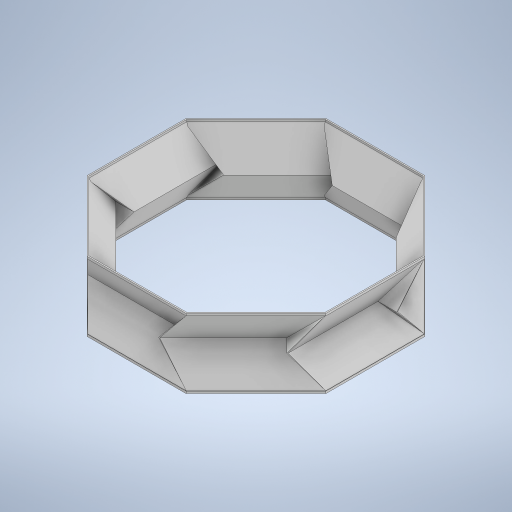
# Autodesk Inventor part: 팔각형 OV-PAM 층 한개
Saved by Autodesk Inventor 2024 (Build 280153000, 153)
## iProperties
Created: 2023-06-16
Part Number: 팔각형 OV-PAM 층 한개
Material: 일반
Document SubType Name: Modeling
Designer: jsw
Density: 1 g/cm^3
Appearance: 기본값
Author: jsw
Autodesk Inventor part; units mm, degrees
ref_plane "YZ Plane" through (0, 0, 0) normal (1, 0, 0) x (0, 1, 0)
ref_plane "XZ Plane" through (0, 0, 0) normal (0, 1, 0) x (-1, 0, 0)
ref_plane "XY Plane" through (0, 0, 0) normal (0, 0, 1) x (1, 0, 0)
sketch "스케치1" plane through (0, 0, 0) normal (0, 1, 0) x (-1, 0, 0)
  line L0 (-65.1838, 27) -> (-27, 65.1838)
  line L1 (-27, 65.1838) -> (27, 65.1838)
  line L2 (27, 65.1838) -> (65.1838, 27)
  line L3 (65.1838, 27) -> (65.1838, -27)
  line L4 (65.1838, -27) -> (27, -65.1838)
  line L5 (27, -65.1838) -> (-27, -65.1838)
  line L6 (-27, -65.1838) -> (-65.1838, -27)
  line L7 (-65.1838, -27) -> (-65.1838, 27)
  line L8 (-27.2485, 65.7838) -> (27.2485, 65.7838)
  line L9 (27.2485, 65.7838) -> (65.7838, 27.2485)
  line L10 (65.7838, 27.2485) -> (65.7838, -27.2485)
  line L11 (65.7838, -27.2485) -> (27.2485, -65.7838)
  line L12 (27.2485, -65.7838) -> (-27.2485, -65.7838)
  line L13 (-27.2485, -65.7838) -> (-65.7838, -27.2485)
  line L14 (-65.7838, -27.2485) -> (-65.7838, 27.2485)
  line L15 (-65.7838, 27.2485) -> (-27.2485, 65.7838)
  point P0 (0, 0)
  point P1 (0, 0)
  point P2 (0, 0)
  dimension "d0" = 54
  dimension "d2" = 0.6
  constraints: 32 end point, 2 coincident, 2 horizontal, 34 other
  measures "d0" distance of L0.end L1.end
  measures "d2" distance between parallel lines of L10 L3
extrude "돌출2" add sketch "스케치1" along normal blind 18 contours L0 L1 L2 L3 L4 L5 L6 L7 | L8 L9 L10 L11 L12 L13 L14 L15
ref_plane "작업 평면2" through (65.7838, 0, 27.2485) normal (-0.8660254, -0.5, 0) x (0, 0, -1)
sketch "스케치3" plane through (65.7838, 0, 27.2485) normal (1, 0, 0) x (0, 0, -1)
  line L0 (0, 0) -> (0, 18) projected
  line L1 (0, 18) -> (54.4971, 18) projected
  line L2 (0, 0) -> (54.4971, 0)
  line L3 (54.4971, 0) -> (54.4971, 18)
  line L4 (54.4971, 18) -> (0, 18)
  line L5 (0, 18) -> (0, 0)
  line L6 (0, 18) -> (-31.1769, 18)
  line L7 (-38.5352, 18) -> (0, 18) projected
  line L8 (0, 0) -> (-31.1769, 18)
  line L9 (54.4971, 18) -> (27.2485, 18)
  line L10 (39.2485, 18) -> (54.4971, 0)
  point P0 (27.2485, 0)
  point P1 (27.2485, 18)
  dimension "d17" = 150
  dimension "d49" = 12
  constraints: 16 end point, 5 midpoint, 2 parallel, 2 point on line, 1 horizontal, 1 perpendicular
  measures "d17" angle of L8 L2
  measures "d49" distance of point (27.249, 18) L10.start
extrude "돌출4" cut sketch "스케치3" against normal up to surface contours L8 L6 L0 | L0 L1 L10 L2 surface through (65.7838, 0, 27.2485) normal (-0.8660254, -0.5, 0)
pattern_circular "원형 패턴1" count 8 over 360 about axis through (0, -10, 0) along (0, 1, 0) of "돌출4"
mirror "미러5" about plane through (0, 18, 0) normal (0, 1, 0) of "돌출2", "돌출4", "원형 패턴1"
sketch "스케치9" plane through (-27.2485, 36, -65.7838) normal (0, 1, 0) x (1, 0, 0)
  line L0 (93.0323, -93.0323) -> (93.0323, -38.5352) projected
  line L1 (93.0323, -38.5352) -> (54.4971, 0) projected
  line L2 (54.4971, 0) -> (0, 0) projected
  line L3 (0, 0) -> (-38.5352, -38.5352) projected
  line L4 (-38.5352, -38.5352) -> (-38.5352, -93.0323) projected
  line L5 (-38.5352, -93.0323) -> (0, -131.5675) projected
  line L6 (0, -131.5675) -> (54.4971, -131.5675) projected
  line L7 (54.4971, -131.5675) -> (93.0323, -93.0323) projected
  point P0 (27.2485, -65.7838)
extrude "돌출8" add sketch "스케치9" along normal blind 1.2
sketch "스케치10" plane through (0, 0, 0) normal (0, -1, 0) x (1, 0, 0)
  line L0 (65.7838, 27.2485) -> (65.7838, -27.2485) projected
  line L1 (27.2485, 65.7838) -> (65.7838, 27.2485) projected
  line L2 (-27.2485, 65.7838) -> (27.2485, 65.7838) projected
  line L3 (-65.7838, 27.2485) -> (-27.2485, 65.7838) projected
  line L4 (-65.7838, -27.2485) -> (-65.7838, 27.2485) projected
  line L5 (-27.2485, -65.7838) -> (-65.7838, -27.2485) projected
  line L6 (27.2485, -65.7838) -> (-27.2485, -65.7838) projected
  line L7 (65.7838, -27.2485) -> (27.2485, -65.7838) projected
  point P0 (0, 0)
extrude "돌출9" add sketch "스케치10" along normal blind 1.2
shell "쉘6" thickness 0.5 removed faces 2 at (-9.0828, 37.2, -21.9279) at (-3.7622, -1.2, -9.0828)
sketch "스케치12" plane through (-27.2485, 37.2, -65.7838) normal (0, 1, 0) x (1, 0, 0)
  line L0 (92.5323, -38.7423) -> (92.5323, -92.8252) projected
  line L1 (92.5323, -92.8252) -> (54.2899, -131.0675) projected
  line L2 (54.2899, -131.0675) -> (0.2071, -131.0675) projected
  line L3 (0.2071, -131.0675) -> (-38.0352, -92.8252) projected
  line L4 (-38.0352, -92.8252) -> (-38.0352, -38.7423) projected
  line L5 (-38.0352, -38.7423) -> (0.2071, -0.5) projected
  line L6 (0.2071, -0.5) -> (54.2899, -0.5) projected
  line L7 (54.2899, -0.5) -> (92.5323, -38.7423) projected
  line L8 (93.0323, -38.5352) -> (54.4971, 0) projected
  line L9 (54.4971, 0) -> (0, 0) projected
  line L10 (0, 0) -> (-38.5352, -38.5352) projected
  line L11 (-38.5352, -38.5352) -> (-38.5352, -93.0323) projected
  line L12 (-38.5352, -93.0323) -> (0, -131.5675) projected
  line L13 (0, -131.5675) -> (54.4971, -131.5675) projected
  line L14 (54.4971, -131.5675) -> (93.0323, -93.0323) projected
  line L15 (93.0323, -93.0323) -> (93.0323, -38.5352) projected
  line L16 (-0.0828, 0.2) -> (54.5799, 0.2)
  line L17 (54.5799, 0.2) -> (93.2323, -38.4524)
  line L18 (93.2323, -38.4524) -> (93.2323, -93.1151)
  line L19 (93.2323, -93.1151) -> (54.5799, -131.7675)
  line L20 (54.5799, -131.7675) -> (-0.0828, -131.7675)
  line L21 (-0.0828, -131.7675) -> (-38.7352, -93.1151)
  line L22 (-38.7352, -93.1151) -> (-38.7352, -38.4524)
  line L23 (-38.7352, -38.4524) -> (-0.0828, 0.2)
  point P0 (27.2485, -65.7838)
  point P1 (27.2485, -65.7838)
  dimension "d50" = 0.2
  constraints: 16 end point, 1 coincident, 1 horizontal, 17 other
  measures "d50" distance between parallel lines of L9 L16
extrude "돌출10" add sketch "스케치12" against normal blind 1.2 contours L16 L17 L18 L19 L20 L21 L22 L23
ref_plane "작업 평면6" through (-27.2485, 18, -65.7838) normal (0, 1, 0) x (1, 0, 0)
mirror "미러8" about plane through (-27.2485, 18, -65.7838) normal (0, 1, 0) of "돌출10"
